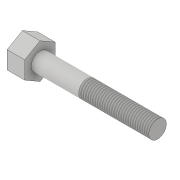
# Autodesk Inventor part: Part1-02
Saved by Autodesk Inventor 2017 (Build 210142000, 142)
## iProperties
Created: 2016-07-21
Part Number: Part1-02
Material: Generic
Document SubType Name: Modeling
Designer: Tutorial Books
Density: 1 g/cm^3
Appearance: Default
Author: Tutorial Books
Autodesk Inventor part; units mm, degrees
ref_plane "YZ Plane" through (0, 0, 0) normal (1, 0, 0) x (0, 1, 0)
ref_plane "XZ Plane" through (0, 0, 0) normal (0, 1, 0) x (-1, 0, 0)
ref_plane "XY Plane" through (0, 0, 0) normal (0, 0, 1) x (1, 0, 0)
sketch "Sketch1" plane through (0, 0, 0) normal (1, 0, 0) x (0, 1, 0)
  circle A0 centre (0, 0) radius 9.525
  dimension "Diameter" = 19.05
  constraints: 1 centre point, 1 coincident
  measures "Diameter" diameter of A0
extrude "Extrusion1" add sketch "Sketch1" along normal blind 127
sketch "Sketch2" plane through (0, 0, 0) normal (1, 0, 0) x (0, 1, 0)
  line L0 (19.05, 0) -> (9.525, -16.4978)
  line L1 (9.525, -16.4978) -> (-9.525, -16.4978)
  line L2 (-9.525, -16.4978) -> (-19.05, 0)
  line L3 (-19.05, 0) -> (-9.525, 16.4978)
  line L4 (-9.525, 16.4978) -> (9.525, 16.4978)
  line L5 (9.525, 16.4978) -> (19.05, 0)
  line L6 (-19.05, 0) -> (19.05, 0) construction
  point P0 (0, 0)
  point P1 (0, 0)
  dimension "Headsize" = 38.1
  constraints: 14 end point, 1 coincident, 1 horizontal, 13 other
  measures "Headsize" distance of L2.end L0.start
extrude "Extrusion2" add sketch "Sketch2" against normal blind 19.05
thread "Thread1" size "3/4-10 UNC" class "2A" standard "ANSI Unified Screw Threads" length 76.2
body "Solid1"
